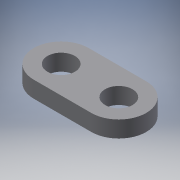
# Autodesk Inventor part: 03連桿15
Saved by Autodesk Inventor 2016 (Build 200138000, 138)
## iProperties
Created: 2017-12-26
Part Number: 03連桿15
Material: 一般
Document SubType Name: Modeling
Designer: user
Density: 1 g/cm^3
Appearance: 預設
Author: user
Autodesk Inventor part; units mm, degrees
ref_plane "YZ Plane" through (0, 0, 0) normal (1, 0, 0) x (0, 1, 0)
ref_plane "XZ Plane" through (0, 0, 0) normal (0, 1, 0) x (-1, 0, 0)
ref_plane "XY Plane" through (0, 0, 0) normal (0, 0, 1) x (1, 0, 0)
sketch "草圖1" plane through (0, 0, 0) normal (0, 0, 1) x (1, 0, 0)
  line L0 (0, 0) -> (10.5, 0) construction
  line L1 (0, -5) -> (10.5, -5)
  line L2 (10.5, 5) -> (0, 5)
  arc A0 (0, 5) -> (0, -5) centre (0, 0) ccw
  arc A1 (10.5, -5) -> (10.5, 5) centre (10.5, 0) ccw
  circle A2 centre (0, 0) radius 2.5
  circle A3 centre (10.5, 0) radius 2.5
  point P0 (5.25, 0)
  dimension "d0" = 10.5
  dimension "d1" = 5
  dimension "d2" = 5
  dimension "d3" = 5
  constraints: 8 end point, 4 centre point, 4 point on circle, 4 tangent, 2 coincident, 1 horizontal, 1 midpoint, 1 parallel
  measures "d0" distance of L0.start L0.end
  measures "d1" radius of A0
  measures "d2" diameter of A2
  measures "d3" diameter of A3
extrude "擠出1" add sketch "草圖1" along normal blind 3
